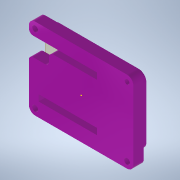
# Autodesk Inventor part: ESP32ParasiteMicroscope_base_v0
Saved by Autodesk Inventor 2022 (Build 260153000, 153)
## iProperties
Created: 2022-02-02
Part Number: ESP32ParasiteMicroscope_base_v0
Material: Generisch
Document SubType Name: Modeling
Designer: diederichbenedict
Density: 1 g/cm^3
Appearance: Glatt - Violett
Author: diederichbenedict
Autodesk Inventor part; units mm, degrees
ref_plane "YZ Plane" through (0, 0, 0) normal (1, 0, 0) x (0, 1, 0)
ref_plane "Arbeitsebene1" through (0, 0, 4) normal (0, 0, 1) x (1, 0, 0)
sketch "Skizze1" plane through (0, 0, 4) normal (0, 0, 1) x (1, 0, 0)
  line L0 (21.8964, 12.5) -> (21.8964, -12.5) construction
  arc A0 (14.8964, -19.5) -> (21.8964, -12.5) centre (14.8964, -12.5) ccw construction
  line L1 (14.8964, -19.5) -> (-23.1036, -19.5) construction
  arc A1 (-30.1036, -12.5) -> (-23.1036, -19.5) centre (-23.1036, -12.5) ccw construction
  line L2 (-30.1036, -12.5) -> (-30.1036, 12.5) construction
  arc A2 (-23.1036, 19.5) -> (-30.1036, 12.5) centre (-23.1036, 12.5) ccw construction
  line L3 (-23.1036, 19.5) -> (14.8964, 19.5) construction
  arc A3 (21.8964, 12.5) -> (14.8964, 19.5) centre (14.8964, 12.5) ccw construction
  line L4 (-26.9233, 19.5) -> (14.8964, 19.5)
  line L5 (14.8964, 19.5) -> (14.8964, -19.4749)
  line L6 (14.8964, -19.4749) -> (-26.9233, -19.4749)
  line L7 (-26.9233, -19.4749) -> (-26.9233, 19.5)
  line L8 (2.5735, 11.7657) -> (-15.3535, 11.7657) construction
  line L9 (2.5735, 13.7657) -> (-15.3535, 13.7657)
  line L10 (-15.3535, 9.7657) -> (2.5735, 9.7657)
  arc A4 (2.5735, 9.7657) -> (2.5735, 13.7657) centre (2.5735, 11.7657) ccw
  arc A5 (-15.3535, 13.7657) -> (-15.3535, 9.7657) centre (-15.3535, 11.7657) ccw
  line L11 (2.4395, -11.3613) -> (-15.3535, -11.3613) construction
  line L12 (2.4395, -9.3613) -> (-15.3535, -9.3613)
  line L13 (-15.3535, -13.3613) -> (2.4395, -13.3613)
  arc A6 (2.4395, -13.3613) -> (2.4395, -9.3613) centre (2.4395, -11.3613) ccw
  arc A7 (-15.3535, -9.3613) -> (-15.3535, -13.3613) centre (-15.3535, -11.3613) ccw
  line L14 (24.9604, -16.4749) -> (24.9604, 19.5) construction
  line L15 (21.9604, 19.5) -> (-22.0396, 19.5) construction
  line L16 (-25.0396, 19.5) -> (-25.0396, -16.4749) construction
  line L17 (-22.0396, -19.4749) -> (24.9604, -19.4749) construction
  line L18 (24.9604, 19.5) -> (14.8964, 19.5)
  line L19 (14.8964, 19.5) -> (14.8964, -19.4749)
  line L20 (14.8964, -19.4749) -> (21.9604, -19.4749)
  line L21 (24.9604, -19.4749) -> (24.9604, 16.5)
  line L22 (-26.9233, 19.5) -> (-25.0396, 19.5)
  line L23 (-25.0396, -19.4749) -> (-26.9233, -19.4749)
  line L24 (-26.9233, -19.4749) -> (-26.9233, 19.5)
  arc A8 (-25.0396, -16.4749) -> (-22.0396, -19.4749) centre (-22.0396, -16.4749) ccw
  arc A9 (-22.0396, 19.5) -> (-25.0396, 16.5) centre (-22.0396, 16.5) ccw
  arc A10 (24.9604, 16.5) -> (21.9604, 19.5) centre (21.9604, 16.5) ccw
  arc A11 (21.9604, -19.4749) -> (24.9604, -16.4749) centre (21.9604, -16.4749) ccw
  line L25 (8.61, 8.7657) -> (-21.39, 8.7657)
  line L26 (-21.39, 8.7657) -> (-21.39, 14.7657)
  line L27 (-21.39, 14.7657) -> (8.61, 14.7657)
  line L28 (8.61, 14.7657) -> (8.61, 8.7657)
  line L29 (8.61, 8.7657) -> (-21.39, 14.7657) construction
  line L30 (-21.39, 8.7657) -> (8.61, 14.7657) construction
  line L31 (8.543, -14.3613) -> (-21.457, -14.3613)
  line L32 (-21.457, -14.3613) -> (-21.457, -8.3613)
  line L33 (-21.457, -8.3613) -> (8.543, -8.3613)
  line L34 (8.543, -8.3613) -> (8.543, -14.3613)
  line L35 (8.543, -14.3613) -> (-21.457, -8.3613) construction
  line L36 (-21.457, -14.3613) -> (8.543, -8.3613) construction
  line L37 (-25.0396, 16.5) -> (-25.0396, -16.4749)
  line L38 (-25.0396, -19.227) -> (-25.0396, -19.4749)
  point P0 (0, 0)
  point P1 (-15.2165, -11.3613)
  point P2 (-6.39, 11.7657)
  point P3 (-6.457, -11.3613)
  point P4 (-24, -18.4749)
  point P5 (33.4901, -16.4749)
  point P6 (-34.4755, 19.5)
  point P7 (-34.4755, -19.4749)
  point P8 (-22.0396, -19.4749)
  dimension "d1" = 4
  dimension "d2" = 4
  dimension "d5" = 3
  dimension "d37" = 30
  dimension "d38" = 6
  dimension "d39" = 6
  dimension "d40" = 30
  dimension "d55" = 50
  constraints: 82 end point, 25 point on circle, 17 tangent, 15 parallel, 12 centre point, 9 point on line, 6 midpoint, 6 perpendicular, 4 horizontal, 3 equal radius, 4 other
  measures "d1" diameter of A5
  measures "d2" diameter of A7
  measures "d5" radius of A8
  measures "d37" distance of L25.start L25.end
  measures "d38" distance of L25.end L26.end
  measures "d39" distance of L31.end L32.end
  measures "d40" distance between parallel lines of L32 L34
  measures "d55" distance between parallel lines of L16 L21
extrude "Extrusion1" add sketch "Skizze1" along normal blind 5 contours L4 L5 L6 A8 L37 A9 | L18 A10 L21 A11 L20 L5 | A4 L10 A5 L9 | A6 L13 A7 L12 | L25 L26 L27 L28 | L31 L32 L33 L34
sketch "Skizze3" plane through (0, 0, 4) normal (0, 0, -1) x (-1, 0, 0)
  line L0 (22.0396, -19.4749) -> (-21.9604, -19.4749) projected
  line L1 (-21.9604, 19.5) -> (22.0396, 19.5) projected
  arc A0 (-21.9604, 19.5) -> (-24.9604, 16.5) centre (-21.9604, 16.5) ccw projected
  line L2 (-24.9604, -16.4749) -> (-24.9604, 16.5) projected
  circle A1 centre (-21.9604, 16.5) radius 1.15
  circle A2 centre (-21.9604, -16.4749) radius 1.4
  circle A3 centre (22.0396, 16.5) radius 1.4
  circle A4 centre (22.0396, -16.4749) radius 1.4
  arc A5 (-24.9604, -16.4749) -> (-21.9604, -19.4749) centre (-21.9604, -16.4749) ccw projected
  line L3 (25.0396, 16.5) -> (25.0396, -16.4749) projected
  arc A6 (25.0396, 16.5) -> (22.0396, 19.5) centre (22.0396, 16.5) ccw projected
  arc A7 (22.0396, -19.4749) -> (25.0396, -16.4749) centre (22.0396, -16.4749) ccw projected
  point P0 (0, 0)
  dimension "d16" = 2.3
  dimension "d17" = 2.8
  dimension "d18" = 2.8
  dimension "d19" = 2.8
  constraints: 4 centre point, 4 coincident
  measures "d16" diameter of A1
  measures "d17" diameter of A2
  measures "d18" diameter of A3
  measures "d19" diameter of A4
extrude "Extrusion3" cut sketch "Skizze3" against normal blind 10 contours A1 | A2 | A3 | A4
sketch "Skizze9" plane through (0, 0, 4) normal (0, 0, -1) x (-1, 0, 0)
  arc A0 (19, -13.5) -> (20, -12.5) centre (19, -12.5) ccw projected
  line L0 (20, -12.5) -> (20, 12.5) projected
  arc A1 (20, 12.5) -> (19, 13.5) centre (19, 12.5) ccw projected
  line L1 (19, 13.5) -> (-19, 13.5) projected
  arc A2 (-19, 13.5) -> (-20, 12.5) centre (-19, 12.5) ccw projected
  line L2 (-20, 12.5) -> (-20, -12.5) projected
  arc A3 (-20, -12.5) -> (-19, -13.5) centre (-19, -12.5) ccw projected
  line L3 (-19, -13.5) -> (19, -13.5) projected
  line L4 (-19, 13.2) -> (19, 13.2)
  arc A4 (19.7, 12.5) -> (19, 13.2) centre (19, 12.5) ccw
  line L5 (19.7, 12.5) -> (19.7, -12.5)
  arc A5 (19, -13.2) -> (19.7, -12.5) centre (19, -12.5) ccw
  line L6 (19, -13.2) -> (-19, -13.2)
  arc A6 (-19.7, -12.5) -> (-19, -13.2) centre (-19, -12.5) ccw
  line L7 (-19.7, -12.5) -> (-19.7, 12.5)
  arc A7 (-19, 13.2) -> (-19.7, 12.5) centre (-19, 12.5) ccw
  line L8 (19, 16.2) -> (-19, 16.2)
  arc A8 (-19, 16.2) -> (-22.7, 12.5) centre (-19, 12.5) ccw
  line L9 (-22.7, 12.5) -> (-22.7, -12.5)
  arc A9 (-22.7, -12.5) -> (-19, -16.2) centre (-19, -12.5) ccw
  line L10 (-19, -16.2) -> (19, -16.2)
  arc A10 (19, -16.2) -> (22.7, -12.5) centre (19, -12.5) ccw
  line L11 (22.7, -12.5) -> (22.7, 12.5)
  arc A11 (22.7, 12.5) -> (19, 16.2) centre (19, 12.5) ccw
  circle A12 centre (-21.9604, 16.5) radius 1.15 projected
  circle A13 centre (22.0396, 16.5) radius 1.4 projected
  circle A14 centre (22.0396, -16.4749) radius 1.4 projected
  circle A15 centre (-21.9604, -16.4749) radius 1.4 projected
  point P0 (0, 0)
  dimension "d46" = 0.3
  dimension "d47" = 3
  constraints: 16 end point, 16 point on circle, 8 centre point, 14 other
  measures "d46" distance between parallel lines of L1 L4
  measures "d47" distance between parallel lines of L4 L8
ref_plane "Arbeitsebene4" through (-20, -13.5, 1.5) normal (0, 0, 1) x (1, 0, 0)
extrude "Extrusion8" add sketch "Skizze9" along normal up to surface (2.5 mm away) contours A11 A13 L11 A10 A14 L10 A9 A15 L9 A8 L8 | A11 A13 | A15 A9 | A10 A14 picked at (21.2445, 15.3819) picked at (-21.1797, -15.4267) picked at (21.1725, -15.4212)
sketch "Skizze10" plane through (19, 16.2, 1.5) normal (0, 0, -1) x (-1, 0, 0)
  arc A0 (38, -29.7) -> (39, -28.7) centre (38, -28.7) ccw projected
  line L0 (39, -28.7) -> (39, -3.7) projected
  arc A1 (39, -3.7) -> (38, -2.7) centre (38, -3.7) ccw projected
  line L1 (38, -2.7) -> (0, -2.7) projected
  arc A2 (0, -2.7) -> (-1, -3.7) centre (0, -3.7) ccw projected
  line L2 (-1, -3.7) -> (-1, -28.7) projected
  arc A3 (-1, -28.7) -> (0, -29.7) centre (0, -28.7) ccw projected
  line L3 (0, -29.7) -> (38, -29.7) projected
  arc A4 (38, -29.7) -> (39, -28.7) centre (38, -28.7) ccw projected
  line L4 (38, -29.7) -> (0, -29.7) projected
  arc A5 (-1, -28.7) -> (0, -29.7) centre (0, -28.7) ccw projected
  line L5 (-1, -28.7) -> (-1, -3.7) projected
  arc A6 (0, -2.7) -> (-1, -3.7) centre (0, -3.7) ccw projected
  line L6 (0, -2.7) -> (38, -2.7) projected
  arc A7 (39, -3.7) -> (38, -2.7) centre (38, -3.7) ccw projected
  line L7 (39, -3.7) -> (39, -28.7) projected
  line L8 (38, 0) -> (0, 0) projected
  arc A8 (0, 0) -> (-3.7, -3.7) centre (0, -3.7) ccw projected
  line L9 (-3.7, -3.7) -> (-3.7, -28.7) projected
  arc A9 (-3.7, -28.7) -> (0, -32.4) centre (0, -28.7) ccw projected
  line L10 (0, -32.4) -> (38, -32.4) projected
  arc A10 (38, -32.4) -> (41.7, -28.7) centre (38, -28.7) ccw projected
  line L11 (41.7, -28.7) -> (41.7, -3.7) projected
  arc A11 (41.7, -3.7) -> (38, 0) centre (38, -3.7) ccw projected
  line L12 (0, -2.4) -> (38, -2.4)
  arc A12 (39.3, -3.7) -> (38, -2.4) centre (38, -3.7) ccw
  line L13 (39.3, -3.7) -> (39.3, -28.7)
  arc A13 (38, -30) -> (39.3, -28.7) centre (38, -28.7) ccw
  line L14 (38, -30) -> (0, -30)
  arc A14 (-1.3, -28.7) -> (0, -30) centre (0, -28.7) ccw
  line L15 (-1.3, -28.7) -> (-1.3, -3.7)
  arc A15 (0, -2.4) -> (-1.3, -3.7) centre (0, -3.7) ccw
  point P0 (19, -16.2)
  dimension "d50" = 0.3
  constraints: 8 end point, 8 point on circle, 4 centre point, 7 other
  measures "d50" distance between parallel lines of L1 L12
ref_plane "Arbeitsebene5" through (-20, -13.5, 0.5) normal (0, 0, -1) x (0, 1, 0)
extrude "Extrusion9" add sketch "Skizze10" along normal up to surface (1 mm away) contours A11 L11 A10 L10 A9 L9 A8 L8
sketch "Skizze11" plane through (19, 16.2, 0.5) normal (0, 0, -1) x (-1, 0, 0)
  arc A0 (-1.3, -28.7) -> (0, -30) centre (0, -28.7) ccw projected
  line L0 (-1.3, -3.7) -> (-1.3, -28.7) projected
  arc A1 (0, -2.4) -> (-1.3, -3.7) centre (0, -3.7) ccw projected
  line L1 (38, -2.4) -> (0, -2.4) projected
  arc A2 (39.3, -3.7) -> (38, -2.4) centre (38, -3.7) ccw projected
  line L2 (39.3, -28.7) -> (39.3, -3.7) projected
  arc A3 (38, -30) -> (39.3, -28.7) centre (38, -28.7) ccw projected
  line L3 (0, -30) -> (38, -30) projected
  line L4 (0, 0) -> (38, 0) projected
  arc A4 (0, 0) -> (-3.7, -3.7) centre (0, -3.7) ccw projected
  line L5 (-3.7, -28.7) -> (-3.7, -3.7) projected
  arc A5 (-3.7, -28.7) -> (0, -32.4) centre (0, -28.7) ccw projected
  line L6 (38, -32.4) -> (0, -32.4) projected
  arc A6 (38, -32.4) -> (41.7, -28.7) centre (38, -28.7) ccw projected
  line L7 (41.7, -3.7) -> (41.7, -28.7) projected
  arc A7 (41.7, -3.7) -> (38, 0) centre (38, -3.7) ccw projected
  line L8 (41.7, -3.7) -> (41.7, -28.7) projected
  line L9 (39.3, -28.7) -> (39.3, -3.7) projected
  line L10 (41.7, -28.7) -> (39.3, -28.7)
  line L11 (39.3, -28.7) -> (39.3, -3.7)
  line L12 (39.3, -3.7) -> (41.7, -3.7)
  line L13 (41.7, -3.7) -> (41.7, -28.7)
  line L14 (39.3, -28.7) -> (36.2612, -28.7)
  line L15 (36.2612, -28.7) -> (36.2612, -3.7)
  line L16 (36.2612, -3.7) -> (39.3, -3.7)
  line L17 (39.3, -3.7) -> (39.3, -28.7)
  point P0 (19, -16.2)
  constraints: 16 end point, 4 parallel, 2 horizontal, 2 perpendicular, 1 point on line
extrude "Extrusion10" cut sketch "Skizze11" against normal up to surface (3.5 mm away) contours L14 L15 L16 L2 | L2 L12 L7 L10
sketch "Sketch12" plane through (0, 0, 9) normal (0, 0, 1) x (1, 0, 0)
  circle A0 centre (21.9604, 16.5) radius 1.15 projected
  line L0 (-25.0396, 16.5) -> (-25.0396, -16.4749) projected
  arc A1 (-25.0396, -16.4749) -> (-22.0396, -19.4749) centre (-22.0396, -16.4749) ccw projected
  line L1 (-22.0396, -19.4749) -> (21.9604, -19.4749) projected
  arc A2 (21.9604, -19.4749) -> (24.9604, -16.4749) centre (21.9604, -16.4749) ccw projected
  line L2 (24.9604, -16.4749) -> (24.9604, 16.5) projected
  arc A3 (24.9604, 16.5) -> (21.9604, 19.5) centre (21.9604, 16.5) ccw projected
  line L3 (21.9604, 19.5) -> (-22.0396, 19.5) projected
  arc A4 (-22.0396, 19.5) -> (-25.0396, 16.5) centre (-22.0396, 16.5) ccw projected
  line L4 (7.5735, -12.7843) -> (-20.3535, -12.7843)
  line L5 (-20.3535, -12.7843) -> (-20.3535, -9.7843)
  line L6 (-20.3535, -9.7843) -> (7.5735, -9.7843)
  line L7 (7.5735, -9.7843) -> (7.5735, -12.7843)
  line L8 (-20.3535, 10.1887) -> (7.5735, 10.1887)
  line L9 (7.5735, 10.1887) -> (7.5735, 13.1887)
  line L10 (7.5735, 13.1887) -> (-20.3535, 13.1887)
  line L11 (-20.3535, 13.1887) -> (-20.3535, 10.1887)
  line L12 (-25.0396, 16.5) -> (-25.0396, -16.4749) projected
  line L13 (-15.3535, 10.1887) -> (-25.0396, 10.1887)
  line L14 (-25.0396, 10.1887) -> (-25.0396, 4.2471)
  line L15 (-25.0396, 4.2471) -> (-15.3535, 4.2471)
  line L16 (-15.3535, 4.2471) -> (-15.3535, 10.1887)
  line L17 (-20.3535, 13.1887) -> (-25.0396, 13.1887)
  line L18 (-25.0396, 13.1887) -> (-25.0396, 10.1887)
  line L19 (-25.0396, 10.1887) -> (-20.3535, 10.1887)
  line L20 (-20.3535, 10.1887) -> (-20.3535, 13.1887)
  point P0 (0, 0)
  point P1 (2.4395, -11.2343)
  point P2 (2.5735, 11.6387)
  point P3 (-15.3535, 11.7657)
  dimension "d56" = 3
  dimension "d57" = 3
  dimension "d58" = 1.55
  dimension "d59" = 1.55
  dimension "d60" = 5
  dimension "d61" = 5
  constraints: 32 end point, 8 parallel, 4 horizontal, 4 perpendicular, 4 point on line, 3 other
  measures "d56" distance between parallel lines of L6 L4
  measures "d57" distance between parallel lines of L10 L8
  measures "d58" distance from line of L4 point (2.44, -11.234)
  measures "d59" distance from line of L10 point (2.574, 11.639)
  measures "d60" distance from line of L9 point (2.574, 11.639)
  measures "d61" distance from line of L11 point (-15.353, 11.766)
extrude "Extrusion11" cut sketch "Sketch12" against normal through all contours L17 L11 L13 L0 | L13 L8 L16 L15 L0 | L10 L9 L8 L11 | L4 L5 L6 L7
fillet "Fillet2" radius 2 4 edges at (-15.3535, 10.1887, 6.5) (-15.3535, 4.2471, 6.5) (-25.0396, 4.2471, 6.5) (-25.0396, 13.1887, 6.5)
sketch "Sketch13" plane through (0, 0, 9) normal (0, 0, 1) x (1, 0, 0)
  point P0 (0, 0)
